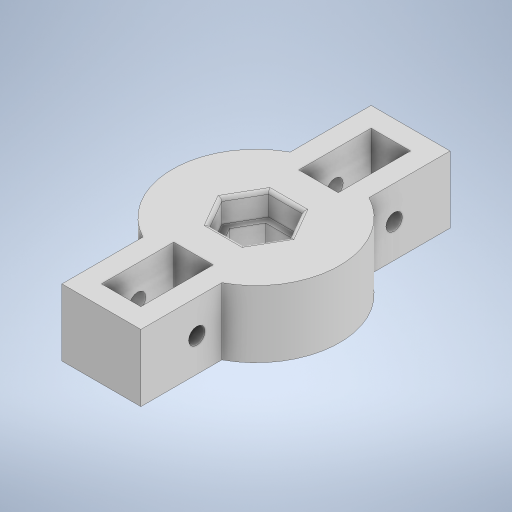
# Autodesk Inventor part: Tensile_test_top_adapter
Saved by Autodesk Inventor 2024 (Build 280153000, 153)
## iProperties
Created: 2023-10-26
Part Number: Tensile_test_top_adapter
Material: 일반
Document SubType Name: Modeling
Designer: jsw
Density: 1 g/cm^3
Appearance: 기본값
Author: jsw
Autodesk Inventor part; units mm, degrees
ref_plane "YZ Plane" through (0, 0, 0) normal (1, 0, 0) x (0, 1, 0)
ref_plane "XZ Plane" through (0, 0, 0) normal (0, 1, 0) x (-1, 0, 0)
ref_plane "XY Plane" through (0, 0, 0) normal (0, 0, 1) x (1, 0, 0)
sketch "스케치1" plane through (0, 0, 0) normal (0, 1, 0) x (-1, 0, 0)
  circle A0 centre (0, 0) radius 12.7
  dimension "d0" = 25.4
  constraints: 1 centre point, 1 coincident
  measures "d0" diameter of A0
extrude "돌출1" add sketch "스케치1" along normal blind 10.16
sketch "스케치2" plane through (0, 10.16, 0) normal (0, 1, 0) x (1, 0, 0)
  circle A0 centre (0, 0) radius 4.5
  line L0 (2.5981, -4.5) -> (-2.5981, -4.5)
  line L1 (-2.5981, -4.5) -> (-5.1962, 0)
  line L2 (-5.1962, 0) -> (-2.5981, 4.5)
  line L3 (-2.5981, 4.5) -> (2.5981, 4.5)
  line L4 (2.5981, 4.5) -> (5.1962, 0)
  line L5 (5.1962, 0) -> (2.5981, -4.5)
  dimension "d3" = 9
  constraints: 12 end point, 2 coincident, 1 centre point, 1 horizontal, 1 tangent, 13 other
  measures "d3" diameter of A0
sketch "스케치3" plane through (0, 0, 0) normal (0, -1, 0) x (1, 0, 0)
  line L0 (-3, 9.5) -> (3, 9.5)
  line L1 (3, 9.5) -> (3, 20.5)
  line L2 (3, 20.5) -> (-3, 20.5)
  line L3 (-3, 20.5) -> (-3, 9.5)
  line L4 (-3, 9.5) -> (3, 20.5) construction
  line L5 (3, 9.5) -> (-3, 20.5) construction
  line L6 (0, 0) -> (5.3002, 0)
  line L7 (-3, -9.5) -> (3, -9.5)
  line L8 (3, -9.5) -> (3, -20.5)
  line L9 (3, -20.5) -> (-3, -20.5)
  line L10 (-3, -20.5) -> (-3, -9.5)
  line L11 (-3, -9.5) -> (3, -20.5) construction
  line L12 (3, -9.5) -> (-3, -20.5) construction
  line L13 (6, 23.5) -> (-6, 23.5)
  line L14 (-6, 23.5) -> (-6, -23.5)
  line L15 (-6, -23.5) -> (6, -23.5)
  line L16 (6, -23.5) -> (6, 23.5)
  line L17 (6, 23.5) -> (-6, -23.5) construction
  line L18 (-6, 23.5) -> (6, -23.5) construction
  circle A0 centre (0, 0) radius 12.7 projected
  point P0 (0, 15)
  point P1 (0, -15)
  point P2 (6, 11.1933)
  point P3 (-6, 11.1933)
  point P4 (-6, -11.1933)
  point P5 (6, -11.1933)
  dimension "d7" = 6
  dimension "d8" = 11
  dimension "d10" = 15
  dimension "d11" = 3
  dimension "d12" = 3
  constraints: 38 end point, 5 symmetric about line, 4 midpoint, 4 parallel, 3 horizontal, 2 perpendicular, 1 vertical alignment
  measures "d7" distance of L2.end L1.end
  measures "d8" distance of L1.end L0.end
  measures "d10" distance of L6.start point (0, 15)
  measures "d11" distance between parallel lines of L2 L13
  measures "d12" distance between parallel lines of L1 L16
extrude "돌출3" add sketch "스케치3" against normal blind 10.16 contours A0 L14 L13 L16 L1 L2 L3 | L3 L2 L1 A0 | A0 L10 L9 L8 L16 L15 L14 | A0 L8 L9 L10
extrude "돌출4" cut sketch "스케치2" against normal blind 8
sketch "스케치4" plane through (0, 2.16, 0) normal (0, 1, 0) x (1, 0, 0)
  line L0 (2.0207, 3.5) -> (4.0415, 0)
  line L1 (4.0415, 0) -> (2.0207, -3.5)
  line L2 (2.0207, -3.5) -> (-2.0207, -3.5)
  line L3 (-2.0207, -3.5) -> (-4.0415, 0)
  line L4 (-4.0415, 0) -> (-2.0207, 3.5)
  line L5 (-2.0207, 3.5) -> (2.0207, 3.5)
  line L6 (-2.5981, 4.5) -> (2.5981, 4.5) projected
  line L7 (2.5981, 4.5) -> (5.1962, 0) projected
  line L8 (-2.5981, 4.5) -> (2.5981, 4.5) projected
  line L9 (-5.1962, 0) -> (-2.5981, 4.5) projected
  line L10 (-2.5981, -4.5) -> (-5.1962, 0) projected
  line L11 (2.5981, -4.5) -> (-2.5981, -4.5) projected
  line L12 (5.1962, 0) -> (2.5981, -4.5) projected
  point P0 (0, 0)
  point P1 (0, 0)
  dimension "d17" = 1
  constraints: 12 end point, 1 coincident, 1 parallel, 13 other
  measures "d17" distance between parallel lines of L6 L5
extrude "돌출5" add sketch "스케치4" along normal blind 4.5
fillet "모깎기2" radius 0.5 6 edges at (3.8971, 10.16, -2.25) (3.8971, 10.16, 2.25) (0, 10.16, -4.5) (0, 10.16, 4.5) (-3.8971, 10.16, 2.25) (-3.8971, 10.16, -2.25)
sketch "스케치6" plane through (0, 10.16, 0) normal (0, 1, 0) x (1, 0, 0)
  line L0 (-3, -9.5) -> (3, -9.5)
  line L1 (3, -9.5) -> (3, -20.5)
  line L2 (3, -20.5) -> (-3, -20.5)
  line L3 (-3, -20.5) -> (-3, -9.5)
  line L4 (-3, -9.5) -> (3, -20.5) construction
  line L5 (3, -9.5) -> (-3, -20.5) construction
  line L6 (-6, -23.5) -> (6, -23.5) projected
  line L7 (6, -23.5) -> (6, -11.1933) projected
  line L8 (2.8868, -5) -> (5.7735, 0) projected
  line L9 (-5.1962, 0) -> (-5.7735, 0) projected
  line L10 (5.7735, 0) -> (-5.7735, 0)
  line L11 (-3, 9.5) -> (3, 9.5)
  line L12 (3, 9.5) -> (3, 20.5)
  line L13 (3, 20.5) -> (-3, 20.5)
  line L14 (-3, 20.5) -> (-3, 9.5)
  line L15 (-3, 9.5) -> (3, 20.5) construction
  line L16 (3, 9.5) -> (-3, 20.5) construction
  line L17 (-6, 23.5) -> (6, 23.5)
  line L18 (6, 23.5) -> (6, 11.1933)
  point P0 (0, 0)
  point P1 (0, -15)
  point P2 (0, 15)
  dimension "d21" = 6
  dimension "d22" = 11
  dimension "d23" = 3
  dimension "d24" = 3
  constraints: 30 end point, 8 symmetric about line, 2 horizontal, 2 midpoint, 2 parallel, 1 perpendicular
  measures "d21" distance of L1.end L2.end
  measures "d22" distance of L0.end L1.end
  measures "d23" distance between parallel lines of L2 L6
  measures "d24" distance between parallel lines of L1 L7
extrude "돌출6" cut sketch "스케치6" against normal blind 10.16
sketch "스케치7" plane through (-6, 0, 11.1933) normal (-1, 0, 0) x (0, 0, 1)
  line L0 (-1.6933, 10.16) -> (9.3067, 10.16) projected
  line L1 (-1.6933, 10.16) -> (-1.6933, 0) projected
  line L2 (9.3067, 0) -> (-1.6933, 0) projected
  line L3 (9.3067, 10.16) -> (9.3067, 0) projected
  line L4 (-31.6933, 10.16) -> (-20.6933, 10.16) projected
  line L5 (-31.6933, 10.16) -> (-31.6933, 0) projected
  line L6 (-20.6933, 0) -> (-31.6933, 0) projected
  line L7 (-20.6933, 10.16) -> (-20.6933, 0) projected
  circle A0 centre (3.8067, 5.08) radius 1.25
  line L8 (-16.1933, 10.16) -> (-11.1933, 10.16) projected
  line L9 (-11.1933, 0) -> (-11.1933, 10.16)
  circle A1 centre (-26.1933, 5.08) radius 1.25
  point P0 (9.3067, 5.08)
  point P1 (3.8067, 0)
  dimension "d27" = 2.5
  constraints: 2 centre point, 2 end point, 2 midpoint, 1 horizontal alignment, 1 perpendicular, 1 symmetric about line, 1 vertical alignment, 1 other
  measures "d27" diameter of A0
extrude "돌출7" cut sketch "스케치7" against normal up to surface (12 mm away) contours A0 | A1
